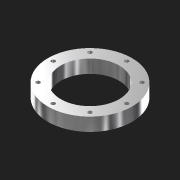
# Autodesk Inventor part: Slewing A
Saved by Autodesk Inventor 2017 (Build 210142000, 142)
## iProperties
Created: 2019-08-28
Part Number: Slewing A
Material: Aluminum 6061
Document SubType Name: Modeling
Designer: Dell
Density: 2.7 g/cm^3
Appearance: Aluminum - Flat
Author: Dell
Autodesk Inventor part; units mm, degrees
ref_plane "YZ Plane" through (0, 0, 0) normal (1, 0, 0) x (0, 1, 0)
ref_plane "XZ Plane" through (0, 0, 0) normal (0, 1, 0) x (-1, 0, 0)
ref_plane "XY Plane" through (0, 0, 0) normal (0, 0, 1) x (1, 0, 0)
sketch "Sketch1" plane through (0, 0, 0) normal (0, 0, 1) x (1, 0, 0)
  circle A0 centre (0, 0) radius 47.5
  circle A1 centre (0, 0) radius 33
  circle A2 centre (41.5, 0) radius 2.25
  circle A3 centre (29.3449, 29.3449) radius 2.25
  circle A4 centre (0, 41.5) radius 2.25
  circle A5 centre (-29.3449, 29.3449) radius 2.25
  circle A6 centre (-41.5, 0) radius 2.25
  circle A7 centre (-29.3449, -29.3449) radius 2.25
  circle A8 centre (0, -41.5) radius 2.25
  circle A9 centre (29.3449, -29.3449) radius 2.25
  dimension "d0" = 95
  dimension "d1" = 66
  dimension "d2" = 4.5
  dimension "d3" = 41.5
  dimension "d6" = 360
  constraints: 10 centre point, 2 coincident, 1 horizontal alignment, 17 other
  measures "d0" diameter of A0
  measures "d1" diameter of A1
  measures "d2" diameter of A2
  measures "d3" distance of point (0, 0) A2.centre
extrude "Extrusion1" add sketch "Sketch1" along normal blind 15
body "Solid1"
